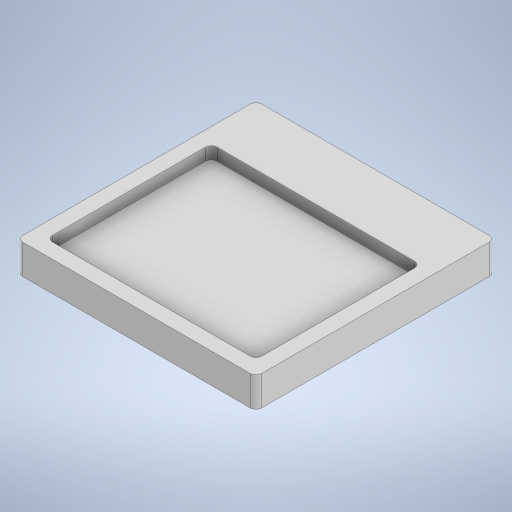
# Autodesk Inventor part: solar-panel-mount
Saved by Autodesk Inventor 2023 (Build 270158000, 158)
## iProperties
Created: 2023-01-30
Part Number: solar-panel-mount
Material: Generic
Document SubType Name: Modeling
Designer: ringl
Density: 1 g/cm^3
Appearance: Default
Author: ringl
Autodesk Inventor part; units mm, degrees
ref_plane "YZ Plane" through (0, 0, 0) normal (1, 0, 0) x (0, 1, 0)
ref_plane "XZ Plane" through (0, 0, 0) normal (0, 1, 0) x (-1, 0, 0)
ref_plane "XY Plane" through (0, 0, 0) normal (0, 0, 1) x (1, 0, 0)
sketch "Sketch1" plane through (0, 0, 0) normal (0, 1, 0) x (-1, 0, 0)
  line L0 (0, 0) -> (80, 0)
  line L1 (80, 0) -> (80, -80)
  line L2 (80, -80) -> (0, -80)
  line L3 (0, -80) -> (0, 0)
  dimension "d0" = 80
  dimension "d1" = 80
  constraints: 8 end point, 2 parallel, 1 horizontal, 1 perpendicular
  measures "d0" distance of L1.end L2.end
  measures "d1" distance of L0.end L1.end
extrude "Extrusion1" add sketch "Sketch1" along normal blind 6
sketch "Sketch2" plane through (0, 6, 0) normal (0, 1, 0) x (1, 0, 0)
  line L0 (-5, 5) -> (-75, 5)
  line L1 (-75, 5) -> (-75, 60)
  line L2 (-75, 60) -> (-5, 60)
  line L3 (-5, 60) -> (-5, 5)
  line L4 (0, 0) -> (0, 80) projected
  line L5 (-80, 0) -> (0, 0) projected
  line L6 (-80, 80) -> (-80, 0) projected
  line L7 (0, 80) -> (-80, 80) projected
  line L8 (-80, 0) -> (0, 0)
  line L9 (0, 0) -> (0, 80)
  line L10 (0, 80) -> (-80, 80)
  line L11 (-80, 80) -> (-80, 0)
  dimension "d8" = 70
  dimension "d9" = 55
  dimension "d10" = 5
  dimension "d11" = 5
  constraints: 16 end point, 4 parallel, 2 horizontal, 2 perpendicular
  measures "d8" distance of L1.end L2.end
  measures "d9" distance of L0.end L1.end
  measures "d10" distance between parallel lines of L4 L3
  measures "d11" distance between parallel lines of L5 L0
extrude "Extrusion2" add sketch "Sketch2" along normal blind 4
fillet "Fillet1" radius 2 4 edges at (-75, 8, -60) (-5, 8, -60) (-5, 8, -5) (-75, 8, -5)
fillet "Fillet2" radius 2 4 edges at (0, 5, 0) (0, 5, -80) (-80, 5, -80) (-80, 5, 0)
body "Solid1"
